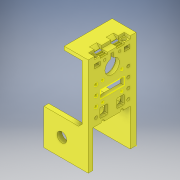
# Autodesk Inventor part: КВ33.044.305 - Крепеж ремня оси Y
Saved by Autodesk Inventor 2019 (Build 230136000, 136)
## iProperties
Created: 2019-08-12
Part Number: КВ33.044.305 - Крепеж ремня оси Y
Material: Пластик АБС
Document SubType Name: Modeling
Designer: Петров Иван
Density: 1.06 g/cm^3
Appearance: Гладкий — желтый
Mass: 19.5226 g
Surface Area: 123.931 cm^2
Volume: 18.4176 cm^3
Author: Петров Иван
Autodesk Inventor part; units mm, degrees
ref_plane "YZ Plane" through (0, 0, 0) normal (1, 0, 0) x (0, 1, 0)
ref_plane "XZ Plane" through (0, 0, 0) normal (0, 1, 0) x (-1, 0, 0)
sketch "Эскиз1" plane through (0, 0, 0) normal (0, 0, 1) x (1, 0, 0)
  line L0 (0, 0) -> (-37, 0)
  line L1 (-37, 0) -> (-37, 30)
  line L2 (-37, 30) -> (0, 30)
  line L3 (0, 30) -> (0, 0)
  line L4 (0, 0) -> (-5, 0)
  line L5 (-5, 0) -> (-5, 80)
  line L6 (-5, 80) -> (0, 80)
  line L7 (0, 80) -> (0, 0)
  dimension "d0" = 37
  dimension "d1" = 30
  dimension "d2" = 5
  dimension "d3" = 80
  constraints: 16 end point, 4 parallel, 2 horizontal, 2 perpendicular
  measures "d0" distance of L1.end L2.end
  measures "d1" distance of L0.end L1.end
  measures "d2" distance of L5.end L6.end
  measures "d3" distance of L4.end L5.end
extrude "Выдавливание1" add sketch "Эскиз1" along normal blind 40
sketch "Эскиз2" plane through (0, 0, 0) normal (1, 0, 0) x (0, 0, -1)
  line L0 (-40, 0) -> (-40, 80) projected
  line L1 (-40, 0) -> (-36, 0)
  line L2 (0, 0) -> (-40, 0) projected
  line L3 (-36, 0) -> (-5, 0)
  line L4 (-5, 0) -> (-5, 31)
  line L5 (-5, 31) -> (-36, 31)
  line L6 (-36, 31) -> (-36, 0)
  dimension "d6" = 4
  dimension "d7" = 31
  dimension "d8" = 31
  constraints: 10 end point, 2 parallel, 1 horizontal, 1 perpendicular, 1 point on line
  measures "d6" distance of L0.start L1.end
  measures "d7" distance of L5.end L4.end
  measures "d8" distance of L4.end L3.end
extrude "Выдавливание2" cut sketch "Эскиз2" against normal blind 44.5
sketch "Эскиз3" plane through (0, 0, 0) normal (1, 0, 0) x (0, 0, -1)
  line L0 (-23.7328, 35.4583) -> (-23.7328, 41.5511)
  arc A0 (-23.7328, 41.5511) -> (-24.6032, 42.4215) centre (-24.6032, 41.5511) ccw
  line L1 (-24.6032, 42.4215) -> (-29.3904, 42.4215)
  line L2 (-23.5, 34.9) -> (-23.5, 45.9)
  line L3 (-23.5, 45.9) -> (-16.5, 45.9)
  line L4 (-16.5, 45.9) -> (-16.5, 34.9)
  line L5 (-16.5, 34.9) -> (-23.5, 34.9)
  line L6 (-19.0049, 77.4) -> (-19.0049, 72.9)
  line L7 (-19.0049, 72.9) -> (-21.0005, 72.9)
  line L8 (-21.0005, 72.9) -> (-21.0005, 77.4)
  line L9 (-21.0005, 77.4) -> (-19.0049, 77.4)
  circle A1 centre (-20, 67.4) radius 6.0225
  line L10 (-30, 55.3) -> (-30, 48.75)
  line L11 (-30, 48.75) -> (-10, 48.75)
  line L12 (-10, 48.75) -> (-10, 55.3)
  line L13 (-10, 55.3) -> (-30, 55.3)
  arc A2 (-23.7328, 41.5511) -> (-24.6032, 42.4215) centre (-24.6032, 41.5511) ccw
  line L14 (-23.7328, 41.5511) -> (-23.7328, 35.4583)
  arc A3 (-24.6032, 34.5879) -> (-23.7328, 35.4583) centre (-24.6032, 35.4583) ccw
  line L15 (-24.6032, 34.5879) -> (-29.3904, 34.5879)
  arc A4 (-30.2608, 35.4583) -> (-29.3904, 34.5879) centre (-29.3904, 35.4583) ccw
  line L16 (-30.2608, 35.4583) -> (-30.2608, 41.5511)
  arc A5 (-29.3904, 42.4215) -> (-30.2608, 41.5511) centre (-29.3904, 41.5511) ccw
  line L17 (-29.3904, 42.4215) -> (-24.6032, 42.4215)
  line L18 (-16.1568, 35.5547) -> (-16.1568, 41.4459)
  arc A6 (-15.3152, 42.2875) -> (-16.1568, 41.4459) centre (-15.3152, 41.4459) ccw
  line L19 (-15.3152, 42.2875) -> (-10.6864, 42.2875)
  arc A7 (-9.8448, 41.4459) -> (-10.6864, 42.2875) centre (-10.6864, 41.4459) ccw
  line L20 (-9.8448, 41.4459) -> (-9.8448, 35.5547)
  arc A8 (-10.6864, 34.7131) -> (-9.8448, 35.5547) centre (-10.6864, 35.5547) ccw
  line L21 (-10.6864, 34.7131) -> (-15.3152, 34.7131)
  arc A9 (-16.1568, 35.5547) -> (-15.3152, 34.7131) centre (-15.3152, 35.5547) ccw
  circle A10 centre (-6.5, 60.9) radius 1.3
  circle A11 centre (-6.5, 52.9) radius 1.3
  circle A12 centre (-6.5, 44.9) radius 1.3
  circle A13 centre (-6.5, 36.9) radius 1.3
  circle A14 centre (-12, 31.4) radius 1.3
  circle A15 centre (-33.5, 36.9) radius 1.3
  circle A16 centre (-33.5, 44.9) radius 1.3
  circle A17 centre (-33.5, 52.9) radius 1.3
  circle A18 centre (-28, 31.4) radius 1.3
  circle A19 centre (-33.5, 60.9) radius 1.3
  circle A20 centre (-12, 45.4) radius 1.05
  circle A21 centre (-28, 45.4) radius 1.05
  circle A22 centre (-12, 61.4) radius 1.05
  circle A23 centre (-28, 61.4) radius 1.05
  circle A24 centre (-13.7371, 75.1697) radius 1.05
  circle A25 centre (-26.2629, 75.1697) radius 1.05
  line L22 (-7.4, 33.6) -> (-7.4, 32.3802)
  arc A26 (-7.4802, 32.3) -> (-7.4, 32.3802) centre (-8.5, 33.4) ccw
  line L23 (-7.4802, 32.3) -> (-8.7, 32.3)
  line L24 (-8.7, 32.3) -> (-8.7, 30)
  line L25 (-8.7, 30) -> (-15.3, 30)
  line L26 (-15.3, 30) -> (-15.3, 32.3)
  line L27 (-15.3, 32.3) -> (-24.7, 32.3)
  line L28 (-24.7, 32.3) -> (-24.7, 30)
  line L29 (-24.7, 30) -> (-31.3, 30)
  line L30 (-31.3, 30) -> (-31.3, 32.3)
  line L31 (-31.3, 32.3) -> (-32.5198, 32.3)
  arc A27 (-32.6, 32.3802) -> (-32.5198, 32.3) centre (-31.5, 33.4) ccw
  line L32 (-32.6, 32.3802) -> (-32.6, 33.6)
  line L33 (-32.6, 33.6) -> (-34.9, 33.6)
  line L34 (-34.9, 33.6) -> (-34.9, 40.2)
  line L35 (-34.9, 40.2) -> (-32.6, 40.2)
  line L36 (-32.6, 40.2) -> (-32.6, 41.6)
  line L37 (-32.6, 41.6) -> (-34.9, 41.6)
  line L38 (-34.9, 41.6) -> (-34.9, 48.2)
  line L39 (-34.9, 48.2) -> (-32.6, 48.2)
  line L40 (-32.6, 48.2) -> (-32.6, 49.6)
  line L41 (-32.6, 49.6) -> (-34.9, 49.6)
  line L42 (-34.9, 49.6) -> (-34.9, 56.2)
  line L43 (-34.9, 56.2) -> (-32.6, 56.2)
  line L44 (-32.6, 56.2) -> (-32.6, 57.6)
  line L45 (-32.6, 57.6) -> (-34.9, 57.6)
  line L46 (-34.9, 57.6) -> (-34.9, 64.2)
  line L47 (-34.9, 64.2) -> (-32.6, 64.2)
  line L48 (-32.6, 64.2) -> (-32.6, 65.4)
  line L49 (-32.6, 65.4) -> (-31.5, 65.4)
  line L50 (-31.5, 65.4) -> (-31.5, 72.9)
  arc A28 (-27, 77.4) -> (-31.5, 72.9) centre (-27, 72.9) ccw
  line L51 (-27, 77.4) -> (-13, 77.4)
  arc A29 (-8.5, 72.9) -> (-13, 77.4) centre (-13, 72.9) ccw
  line L52 (-8.5, 72.9) -> (-8.5, 65.4)
  line L53 (-8.5, 65.4) -> (-7.4, 65.4)
  line L54 (-7.4, 65.4) -> (-7.4, 64.2)
  line L55 (-7.4, 64.2) -> (-5.1, 64.2)
  line L56 (-5.1, 64.2) -> (-5.1, 57.6)
  line L57 (-5.1, 57.6) -> (-7.4, 57.6)
  line L58 (-7.4, 57.6) -> (-7.4, 56.2)
  line L59 (-7.4, 56.2) -> (-5.1, 56.2)
  line L60 (-5.1, 56.2) -> (-5.1, 49.6)
  line L61 (-5.1, 49.6) -> (-7.4, 49.6)
  line L62 (-7.4, 49.6) -> (-7.4, 48.2)
  line L63 (-7.4, 48.2) -> (-5.1, 48.2)
  line L64 (-5.1, 48.2) -> (-5.1, 41.6)
  line L65 (-5.1, 41.6) -> (-7.4, 41.6)
  line L66 (-7.4, 41.6) -> (-7.4, 40.2)
  line L67 (-7.4, 40.2) -> (-5.1, 40.2)
  line L68 (-5.1, 40.2) -> (-5.1, 33.6)
  line L69 (-5.1, 33.6) -> (-7.4, 33.6)
  circle A30 centre (-20, 67.4) radius 1.3687
  line L70 (-5.1, 64.2) -> (-5.1, 57.6)
  line L71 (-5, 31) -> (-36, 31) projected
  line L72 (-20.5, 31) -> (-20.5, 68.4)
  line L73 (-26.9968, 42.4215) -> (-26.9968, 34.5879)
  line L74 (-30.2608, 38.5047) -> (-23.7328, 38.5047)
  line L75 (-13.0008, 42.2875) -> (-13.0008, 34.7131)
  line L76 (-16.1568, 38.5003) -> (-9.8448, 38.5003)
  point P0 (0, 0)
  point P1 (-20, 67.4)
  dimension "d11" = 37.4
  constraints: 152 end point, 31 centre point, 26 point on circle, 9 midpoint, 1 vertical
  measures "d11" distance of L72.start L72.end
extrude "Выдавливание3" cut sketch "Эскиз3" against normal blind 44.5 contours A3 L15 L73 L74 L0 | L74 L73 L1 A0 L0 | L74 L16 A5 L1 L73 | L73 L15 A4 L16 L74 | L72 L13 L12 L11 | L11 L10 L13 L72 | A1 L8 L7 L6 | L71 A14 | A14 L71 | L71 A18 | A18 L71 | A1 L6 L7 L8 | L8 L9 L6 A1 | L18 L76 L75 L21 A9 | L18 A6 L19 L75 L76 | L76 L20 A8 L21 L75 | L75 L19 A7 L20 L76 | A10 | A11 | A12 | A13 | A15 | A16 | A17 | A19 | A20 | A21 | A22 | A23 | A24 | A25 | A30
sketch "Эскиз4" plane through (0, 0, 40) normal (0, 0, 1) x (1, 0, 0)
  line L0 (-37, 30) -> (-37, 0) projected
  line L1 (-37, 15) -> (-22, 15)
  circle A0 centre (-22, 15) radius 4.1
  point P0 (0, 0)
  dimension "d14" = 15
  dimension "d15" = 8.2
  constraints: 2 end point, 1 centre point, 1 coincident, 1 horizontal, 1 midpoint
  measures "d14" distance of L1.start L1.end
  measures "d15" diameter of A0
extrude "Выдавливание4" cut sketch "Эскиз4" against normal blind 44.5
chamfer "Фаска1" distance 3 angle 45 2 edges at (-5, 30, 2.5) (-5, 30, 38)
chamfer "Фаска2" distance 2 angle 45 21 edges at (-5, 61.3775, 19.9973) (-5, 48.75, 20) (-5, 52.025, 10) (-5, 55.3, 20) (-5, 52.025, 30) (-5, 34.7131, 13.0008) (-5, 34.9596, 10.0913) (-5, 38.5003, 9.8448) (-5, 42.041, 10.0913) (-5, 42.2875, 13.0008) (-5, 42.041, 15.9103) (-5, 38.5003, 16.1568) (-5, 34.9596, 15.9103) (-5, 38.5047, 23.7328) (-5, 42.1665, 23.9878) (-5, 42.4215, 26.9968) (-5, 42.1665, 30.0059) (-5, 38.5047, 30.2608) (-5, 34.8428, 30.0059) (-5, 34.5879, 26.9968) (-5, 34.8428, 23.9878)
sketch "Эскиз10" plane through (-5, 80, 0) normal (0, 1, 0) x (1, 0, 0)
  line L0 (5, 0) -> (0, 0) projected
  line L1 (-3, -40) -> (-32, -40) projected
  line L2 (5, 0) -> (-15, 0)
  line L3 (-15, 0) -> (-15, -40)
  line L4 (-15, -40) -> (5, -40)
  line L5 (5, -40) -> (5, 0)
  dimension "d47" = 20
  constraints: 8 end point, 2 parallel, 1 horizontal, 1 perpendicular, 1 point on line
  measures "d47" distance of L4.end L3.end
extrude "Выдавливание9" add sketch "Эскиз10" along normal blind 2 and the other way blind 1
sketch "Эскиз11" plane through (-5, 82, 0) normal (0, 1, 0) x (1, 0, 0)
  line L0 (5, 0) -> (5, -5) projected
  line L1 (-32, -40) -> (5, -40) projected
  line L2 (5, 0) -> (5, -40)
  line L3 (5, -40) -> (5, -13)
  line L4 (5, -13) -> (1.871, -13)
  line L5 (5, -13.9775) -> (5, -26.0225) projected
  line L6 (-1.258, -16) -> (5, -16)
  line L7 (5, -16) -> (5, -10)
  line L8 (5, -10) -> (-1.258, -10)
  line L9 (-1.258, -10) -> (-1.258, -16)
  line L10 (-1.258, -16) -> (5, -10) construction
  line L11 (5, -16) -> (-1.258, -10) construction
  point P0 (5, -19.0049)
  point P1 (5, -21.0005)
  dimension "d52" = 27
  dimension "d55" = 6
  constraints: 18 end point, 2 midpoint, 2 parallel, 2 perpendicular, 2 point on line, 1 horizontal, 1 vertical
  measures "d52" distance of L1.end L3.end
  measures "d55" distance of L8.end L6.start
extrude "Выдавливание10" cut sketch "Эскиз11" against normal blind 4.25
chamfer "Фаска3" distance 2.75 angle 45 1 edges at (-6.258, 82, 13)
sketch "Эскиз12" plane through (-5, 77.75, 0) normal (0, 1, 0) x (1, 0, 0)
  line L0 (0, -10) -> (5, -10) projected
  line L1 (5, -16) -> (-4.008, -16) projected
  line L2 (5, -10) -> (3.86, -10)
  line L3 (3.86, -10) -> (3.86, -16)
  line L4 (3.86, -16) -> (5, -16)
  line L5 (5, -16) -> (5, -10)
  line L6 (1.86, -10) -> (3, -10)
  line L7 (3, -10) -> (3, -16)
  line L8 (3, -16) -> (1.86, -16)
  line L9 (1.86, -16) -> (1.86, -10)
  line L10 (2.43, -10) -> (2.43, -17.6585)
  line L11 (4.43, -10) -> (4.43, -17.5329)
  line L12 (-0.14, -10) -> (1, -10)
  line L13 (1, -10) -> (1, -16)
  line L14 (1, -16) -> (-0.14, -16)
  line L15 (-0.14, -16) -> (-0.14, -10)
  line L16 (0.43, -10) -> (0.43, -17.8295)
  point P0 (5, 0)
  dimension "d59" = 1.14
  dimension "d60" = 1.14
  dimension "d61" = 2
  dimension "d62" = 1.14
  dimension "d63" = 2
  constraints: 30 end point, 6 parallel, 5 point on line, 4 perpendicular, 3 horizontal, 3 midpoint, 2 vertical
  measures "d59" distance of L4.end L3.end
  measures "d60" distance of L7.end L8.end
  measures "d61" distance between parallel lines of L11 L10
  measures "d62" distance of L13.end L14.end
  measures "d63" distance between parallel lines of L16 L10
extrude "Выдавливание11" add sketch "Эскиз12" along normal blind 0.6 contours L0 L16 L1 L15 L12 | L0 L13 L1 L16 | L0 L10 L1 L9 | L0 L7 L1 L10 | L0 L11 L1 L3 | L0 L5 L1 L11
ref_plane "РабПлоскость1" through (0, 77.4, 20.0027) normal (0, 0, 1) x (1, 0, 0)
mirror "Зеркальное отражение1" about plane through (0, 77.4, 20.0027) normal (0, 0, 1) of "Выдавливание11", "Выдавливание10", "Фаска3"
chamfer "Фаска4" distance 0.2 angle 45 12 edges at (-5.14, 78.35, 13) (-4, 78.35, 13) (-3.14, 78.35, 13) (-1.14, 78.35, 13) (-2, 78.35, 13) (0, 78.35, 13) (0, 78.35, 27.0054) (-2, 78.35, 27.0054) (-3.14, 78.35, 27.0054) (-1.14, 78.35, 27.0054) (-4, 78.35, 27.0054) (-5.14, 78.35, 27.0054)
sketch "Эскиз13" plane through (-5, 82, 0) normal (0, 1, 0) x (1, 0, 0)
  line L0 (-0.14, -30.0054) -> (-0.14, -24.0054) projected
  line L1 (-0.14, -30.0054) -> (-0.14, -35.0054)
  line L2 (5, -10) -> (5, 0) projected
  line L3 (5, -10) -> (5, -5)
  line L4 (5, -5) -> (0, -5) projected
  line L5 (0, -34.8) -> (0, -32.2) projected
  line L6 (5, -5) -> (0, -5)
  line L7 (0, -5) -> (0, -34.8)
  line L8 (0, -34.8) -> (5, -34.8)
  line L9 (5, -34.8) -> (5, -5)
  dimension "d69" = 5
  dimension "d70" = 5
  constraints: 12 end point, 2 parallel, 1 horizontal, 1 midpoint, 1 perpendicular, 1 vertical
  measures "d69" distance of L0.start L1.end
  measures "d70" distance of L2.start L3.end
extrude "Выдавливание12" cut sketch "Эскиз13" against normal blind 2.4
sketch "Эскиз14" plane through (-5, 79.6, 0) normal (0, 1, 0) x (1, 0, 0)
  line L0 (0, -34.8) -> (0, -32.2608) projected
  line L1 (5, -32.2) -> (0.0608, -32.2) projected
  line L2 (0, -34.8) -> (2.5304, -34.8)
  line L3 (2.5304, -34.8) -> (2.5304, -32.2)
  line L4 (2.5304, -32.2) -> (0, -32.2)
  line L5 (0, -32.2) -> (0, -34.8)
  circle A0 centre (2.5304, -32.2) radius 1.75
  point P0 (5, 0)
  dimension "d73" = 3.5
  constraints: 8 end point, 2 parallel, 1 centre point, 1 coincident, 1 horizontal, 1 midpoint, 1 perpendicular
  measures "d73" diameter of A0
extrude "Выдавливание13" cut sketch "Эскиз14" against normal blind 5 contours A0 L1 L3 | L3 L1 A0 | L1 A0
sketch "Эскиз15" plane through (0, 0, 36) normal (1, 0, 0) x (0, 0, -1)
  line L0 (5.9946, 79.6) -> (1.2, 79.6) projected
  line L1 (3.5973, 79.6) -> (3.5973, 74.6)
  line L2 (1.2473, 72.95) -> (5.9473, 72.95)
  line L3 (5.9473, 72.95) -> (5.9473, 76.25)
  line L4 (5.9473, 76.25) -> (1.2473, 76.25)
  line L5 (1.2473, 76.25) -> (1.2473, 72.95)
  line L6 (1.2473, 72.95) -> (5.9473, 76.25) construction
  line L7 (5.9473, 72.95) -> (1.2473, 76.25) construction
  point P0 (36, 0)
  dimension "d76" = 5
  dimension "d77" = 4.7
  dimension "d78" = 3.3
  constraints: 14 end point, 3 midpoint, 2 parallel, 1 horizontal, 1 perpendicular, 1 vertical
  measures "d76" distance of L1.start L1.end
  measures "d77" distance of L4.end L3.end
  measures "d78" distance of L3.end L2.end
extrude "Выдавливание14" cut sketch "Эскиз15" against normal blind 8.75
mirror "Зеркальное отражение2" about plane through (0, 77.4, 20.0027) normal (0, 0, 1) of "Выдавливание14", "Выдавливание13"
sketch "Эскиз16" plane through (-5, 79.6, 0) normal (0, 1, 0) x (1, 0, 0)
  circle A0 centre (2.5304, -32.2) radius 1.75 projected
  line L0 (0, -30.0054) -> (5, -30.0054) projected
  line L1 (0, -34.8) -> (0, -30.0054) projected
  line L2 (5, -34.8) -> (0, -34.8) projected
  line L3 (5, -30.0054) -> (5, -34.8) projected
  line L4 (0, -16) -> (5, -16) projected
  line L5 (0, -24.0054) -> (0, -16) projected
  line L6 (5, -24.0054) -> (0, -24.0054) projected
  line L7 (5, -16) -> (5, -24.0054) projected
  circle A1 centre (2.5304, -7.8054) radius 1.75 projected
  line L8 (5, -10) -> (0, -10) projected
  line L9 (5, -5) -> (5, -10) projected
  line L10 (0, -5) -> (5, -5) projected
  line L11 (0, -10) -> (0, -5) projected
  point P0 (5, 0)
sketch "Эскиз17" plane through (0, 0, 36) normal (1, 0, 0) x (0, 0, -1)
  circle A0 centre (2.5, 60.9) radius 1.3 projected
  circle A1 centre (8, 61.4) radius 1.05 projected
  circle A2 centre (2.5, 52.9) radius 1.3 projected
  circle A3 centre (2.5, 44.9) radius 1.3 projected
  circle A4 centre (8, 45.4) radius 1.05 projected
  circle A5 centre (24, 45.4) radius 1.05 projected
  circle A6 centre (24, 61.4) radius 1.05 projected
  line L0 (6, 55.3) -> (26, 55.3) projected
  line L1 (6, 48.75) -> (6, 55.3) projected
  line L2 (26, 48.75) -> (6, 48.75) projected
  line L3 (26, 55.3) -> (26, 48.75) projected
  point P0 (36, 0)
